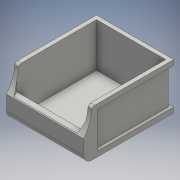
# Autodesk Inventor part: box
Saved by Autodesk Inventor 2016 (Build 200138000, 138)
## iProperties
Created: 2015-09-09
Part Number: box
Material: Generic
Document SubType Name: Modeling
Designer: oscar
Density: 1 g/cm^3
Appearance: Default
Author: oscar
Autodesk Inventor part; units mm, degrees
ref_plane "YZ Plane" through (0, 0, 0) normal (1, 0, 0) x (0, 1, 0)
ref_plane "XZ Plane" through (0, 0, 0) normal (0, 1, 0) x (-1, 0, 0)
sketch "Sketch1" plane through (0, 0, 0) normal (0, 0, 1) x (1, 0, 0)
  line L0 (0, 0) -> (-137, 0)
  line L1 (-137, 0) -> (-137, 160)
  line L2 (-137, 160) -> (0, 160)
  line L3 (0, 160) -> (0, 0)
  dimension "d0" = 137
  dimension "d1" = 160
  constraints: 8 end point, 2 parallel, 1 horizontal, 1 perpendicular
  measures "d0" distance of L1.end L2.end
  measures "d1" distance of L0.end L1.end
extrude "Extrusion1" add sketch "Sketch1" along normal blind 82
sketch "Sketch2" plane through (0, 0, 82) normal (0, 0, 1) x (1, 0, 0)
  line L0 (-7, 11) -> (-130, 11)
  line L1 (-130, 11) -> (-130, 153)
  line L2 (-130, 153) -> (-7, 153)
  line L3 (-7, 153) -> (-7, 11)
  line L4 (-137, 160) -> (-137, 0) projected
  line L5 (0, 0) -> (0, 160) projected
  line L6 (0, 160) -> (-137, 160) projected
  line L7 (-137, 0) -> (0, 0) projected
  dimension "d4" = 7
  dimension "d5" = 7
  dimension "d6" = 7
  dimension "d7" = 11
  constraints: 8 end point, 2 parallel, 1 horizontal, 1 perpendicular
  measures "d4" distance between parallel lines of L4 L1
  measures "d5" distance between parallel lines of L5 L3
  measures "d6" distance between parallel lines of L6 L2
  measures "d7" distance between parallel lines of L7 L0
extrude "Extrusion2" cut sketch "Sketch2" against normal blind 78 contours L0 L1 L2 L3
sketch "Sketch3" plane through (0, 0, 82) normal (0, 0, 1) x (1, 0, 0)
  line L0 (-7, 11) -> (-130, 11) projected
  line L1 (-130, 11) -> (-123.6491, 0)
  line L2 (0, 0) -> (-137, 0) projected
  line L3 (-130, 11) -> (-117.2983, 11) construction
  line L4 (-7, 11) -> (-13.3509, 0)
  line L5 (-7, 11) -> (5.7017, 11) construction
  line L6 (-13.3509, 0) -> (-123.6491, 0)
  line L7 (-130, 11) -> (-7, 11)
  dimension "d10" = 60
  dimension "d11" = 120
  constraints: 12 end point, 3 horizontal, 2 equal length, 2 point on line, 1 collinear
  measures "d10" angle of L1 L3
  measures "d11" angle of L4 L5
extrude "Extrusion3" cut sketch "Sketch3" against normal blind 40
sketch "Sketch4" plane through (-137, 0, 0) normal (-1, 0, 0) x (0, 0, 1)
  line L0 (73, 160) -> (9, 160)
  line L1 (9, 160) -> (9, 25)
  line L2 (9, 25) -> (73, 25)
  line L3 (73, 25) -> (73, 160)
  line L4 (82, 160) -> (82, 0) projected
  line L5 (0, 0) -> (0, 160) projected
  line L6 (0, 160) -> (82, 160) projected
  line L7 (0, 0) -> (82, 0) projected
  dimension "d14" = 9
  dimension "d15" = 9
  dimension "d16" = 0
  dimension "d17" = 25
  constraints: 8 end point, 2 parallel, 1 horizontal, 1 perpendicular
  measures "d14" distance between parallel lines of L4 L3
  measures "d15" distance between parallel lines of L5 L1
  measures "d16" distance between parallel lines of L6 L0
  measures "d17" distance between parallel lines of L7 L2
extrude "Extrusion4" cut sketch "Sketch4" against normal blind 5 contours L3 L2 L1 L0
ref_plane "Work Plane1" through (-68.5, 0, 0) normal (1, 0, 0) x (0, 0, -1)
mirror "Mirror1" about plane through (-68.5, 0, 0) normal (1, 0, 0) of "Extrusion4"
sketch "Sketch5" plane through (-137, 160, 0) normal (0, 1, 0) x (1, 0, 0)
  line L0 (137, -73) -> (132, -73) projected
  line L1 (5, -73) -> (5, -9) projected
  line L2 (132, -73) -> (5, -73)
  line L3 (5, -73) -> (5, -9)
  line L4 (5, -9) -> (132, -9)
  line L5 (132, -9) -> (132, -73)
  point P0 (137, 0)
  constraints: 8 end point, 2 parallel, 1 horizontal, 1 perpendicular
extrude "Extrusion5" cut sketch "Sketch5" against normal blind 5
fillet "Fillet1" radius 15 1 edges at (-68.5, 11, 4)
fillet "Fillet2" radius 15 1 edges at (-68.5, 0, 0)
sketch "Sketch6" plane through (-137, 0, 82) normal (-1, 0, 0) x (0, 0, 1)
  circle A0 centre (0, -50) radius 65
  line L0 (-67, 0) -> (0, 0) projected
  line L1 (0, 160) -> (0, 0) projected
  point P0 (-82, 0)
  dimension "d24" = 130
  dimension "d25" = 50
  dimension "d26" = 0
  constraints: 1 centre point
  measures "d24" diameter of A0
  measures "d25" distance from line of L0 A0.centre
  measures "d26" distance from line of L1 A0.centre
extrude "Extrusion6" cut sketch "Sketch6" against normal through all
fillet "Fillet3" radius 5 2 edges at (-133.5, 15, 82) (-3.5, 15, 82)
body "Solid1"
